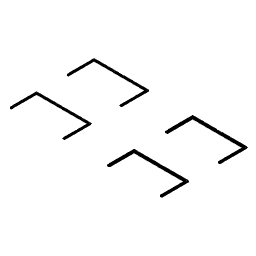
V1_V2_Panels (Autodesk Fusion 360 design; units mm, degrees)
Autodesk Fusion 360 part; units mm, degrees
note: some values were not read from the file. Chosen so that the rebuilt part matches the saved one: which bodies a step acts on; which face or edge a step refers to. Set by a fixed rule: which sketch regions a step uses.
(part 1 of 2)
sketch "Master Sketch" plane through (0, 0, 0) normal (0, 0, 1) x (1, 0, 0)
  line L0 (-121.0378, 68.2273) -> (387.1017, 68.2273)
  line L1 (389.1017, 66.2273) -> (389.1017, -187.8424)
  line L2 (-123.0378, -187.8424) -> (-123.0378, 66.2273)
  line L3 (-110.0378, -187.8424) -> (376.1017, -187.8424)
  line L4 (376.1017, -187.8424) -> (376.1017, 55.2273)
  line L5 (376.1017, 55.2273) -> (-110.0378, 55.2273)
  line L6 (-110.0378, 55.2273) -> (-110.0378, -187.8424)
  line L7 (133.0319, 68.2273) -> (133.0319, -187.8424)
  circle A0 centre (-98.0378, 64.1773) radius 3.05
  circle A1 centre (-73.0378, 58.2273) radius 1.7
  circle A2 centre (-73.0378, 58.2273) radius 2.95
  circle A3 centre (4.997, 58.2273) radius 2.95
  circle A4 centre (4.997, 58.2273) radius 1.7
  circle A5 centre (83.0319, 58.2273) radius 2.95
  circle A6 centre (83.0319, 58.2273) radius 1.7
  line L8 (153.0319, 68.2273) -> (113.0319, 68.2273) construction
  arc A7 (111.0319, 68.2273) -> (113.0319, 66.2273) centre (113.0319, 68.2273) ccw
  line L9 (113.0319, 66.2273) -> (133.0319, 66.2273)
  line L10 (153.0319, 68.2273) -> (113.0319, 68.2273) construction
  arc A8 (-121.0378, 68.2273) -> (-123.0378, 66.2273) centre (-121.0378, 66.2273) ccw
  arc A9 (389.1017, 66.2273) -> (387.1017, 68.2273) centre (387.1017, 66.2273) ccw
  line L11 (83.0319, 58.2273) -> (-73.0378, 58.2273) construction
  circle A10 centre (-143, 12) radius 3.05
  circle A11 centre (-143, -4) radius 1.7
  circle A12 centre (-143, -4) radius 2.95
  circle A13 centre (-118.9878, 43.2273) radius 3.05
  circle A14 centre (-113.0378, 18.2273) radius 1.7
  circle A15 centre (-113.0378, 18.2273) radius 2.95
  circle A16 centre (-113.0378, -59.8075) radius 1.7
  circle A17 centre (-113.0378, -59.8075) radius 2.95
  circle A18 centre (-113.0378, -137.8424) radius 1.7
  circle A19 centre (-113.0378, -137.8424) radius 2.95
  line L12 (-113.0378, 18.2273) -> (-113.0378, -137.8424) construction
  line L13 (-121.0378, -187.8424) -> (-121.0378, -167.8424)
  arc A20 (-121.0378, -167.8424) -> (-123.0378, -165.8424) centre (-123.0378, -167.8424) ccw
  line L14 (-123.0378, -187.8424) -> (-123.0378, -167.8424) construction
  line L15 (387.1017, -187.8424) -> (387.1017, -167.8424)
  line L16 (389.1017, -187.8424) -> (389.1017, -167.8424) construction
  arc A21 (389.1017, -165.8424) -> (387.1017, -167.8424) centre (389.1017, -167.8424) ccw
  circle A22 centre (379.1017, -59.8075) radius 2.95
  circle A23 centre (379.1017, -59.8075) radius 1.7
  circle A24 centre (379.1017, -137.8424) radius 1.7
  circle A25 centre (379.1017, -137.8424) radius 2.95
  circle A26 centre (379.1017, 18.2273) radius 1.7
  circle A27 centre (379.1017, 18.2273) radius 2.95
  circle A28 centre (339.1017, 58.2273) radius 1.7
  circle A29 centre (261.0668, 58.2273) radius 2.95
  arc A30 (153.0319, 66.2273) -> (155.0319, 68.2273) centre (153.0319, 68.2273) ccw
  line L17 (183.0319, 58.2273) -> (339.1017, 58.2273) construction
  circle A31 centre (183.0319, 58.2273) radius 2.95
  circle A32 centre (183.0319, 58.2273) radius 1.7
  circle A33 centre (339.1017, 58.2273) radius 2.95
  circle A34 centre (261.0668, 58.2273) radius 1.7
  line L18 (153.0319, 66.2273) -> (133.0319, 66.2273)
  line L19 (389.1017, -187.8424) -> (133.0319, -187.8424)
  line L20 (-110.0378, -187.8424) -> (-123.0378, -187.8424)
  circle A35 centre (-29.3479, 64.1773) radius 3.05
  circle A36 centre (39.342, 64.1773) radius 3.05
  circle A37 centre (-143, 12) radius 3.05
  circle A38 centre (108.0319, 64.1773) radius 3.05
  circle A39 centre (-118.9878, -25.4626) radius 3.05
  circle A40 centre (-118.9878, -94.1525) radius 3.05
  circle A41 centre (-118.9878, -162.8424) radius 3.05
  circle A42 centre (385.0517, -162.8424) radius 3.05
  circle A43 centre (385.0517, -94.1525) radius 3.05
  circle A44 centre (385.0517, -25.4626) radius 3.05
  circle A45 centre (364.1017, 64.1773) radius 3.05
  circle A46 centre (385.0517, 43.2273) radius 3.05
  circle A47 centre (226.7218, 64.1773) radius 3.05
  circle A48 centre (295.4117, 64.1773) radius 3.05
  circle A49 centre (158.0319, 64.1773) radius 3.05
  line L21 (813.9622, -187.8424) -> (1302.1017, -187.8424)
  line L22 (803.9622, 68.2273) -> (1312.1017, 68.2273)
  circle A50 centre (1310.0517, 43.2273) radius 3.05
  circle A51 centre (1083.0319, 64.1773) radius 3.05
  line L23 (1078.0319, 66.2273) -> (1058.0319, 66.2273)
  arc A52 (1078.0319, 66.2273) -> (1080.0319, 68.2273) centre (1078.0319, 68.2273) ccw
  arc A53 (803.9622, -167.8424) -> (801.9622, -165.8424) centre (801.9622, -167.8424) ccw
  circle A54 centre (1151.7218, 64.1773) radius 3.05
  circle A55 centre (806.0122, 43.2273) radius 3.05
  circle A56 centre (1220.4117, 64.1773) radius 3.05
  circle A57 centre (826.9622, 64.1773) radius 3.05
  circle A58 centre (1289.1017, 64.1773) radius 3.05
  line L24 (1301.1017, 56.2273) -> (814.9622, 56.2273)
  line L25 (1314.1017, -187.8424) -> (1058.0319, -187.8424)
  line L26 (1314.1017, 66.2273) -> (1314.1017, -187.8424)
  line L27 (813.9622, 55.2273) -> (813.9622, -187.8424)
  line L28 (1058.0319, 68.2273) -> (1058.0319, -187.8424)
  line L29 (801.9622, -187.8424) -> (801.9622, 66.2273)
  line L30 (1302.1017, -187.8424) -> (1302.1017, 55.2273)
  line L31 (1078.0319, 68.2273) -> (1038.0319, 68.2273) construction
  circle A59 centre (964.342, 64.1773) radius 3.05
  line L32 (803.9622, -187.8424) -> (803.9622, -167.8424)
  line L33 (1078.0319, 68.2273) -> (1038.0319, 68.2273) construction
  circle A60 centre (895.6521, 64.1773) radius 3.05
  circle A61 centre (1033.0319, 64.1773) radius 3.05
  line L34 (801.9622, -187.8424) -> (801.9622, -167.8424) construction
  arc A62 (1036.0319, 68.2273) -> (1038.0319, 66.2273) centre (1038.0319, 68.2273) ccw
  arc A63 (803.9622, 68.2273) -> (801.9622, 66.2273) centre (803.9622, 66.2273) ccw
  circle A64 centre (806.0122, -162.8424) radius 3.05
  circle A65 centre (806.0122, -94.1525) radius 3.05
  line L35 (813.9622, -187.8424) -> (801.9622, -187.8424)
  circle A66 centre (806.0122, -25.4626) radius 3.05
  arc A67 (1314.1017, -165.8424) -> (1312.1017, -167.8424) centre (1314.1017, -167.8424) ccw
  line L36 (1038.0319, 66.2273) -> (1058.0319, 66.2273)
  arc A68 (1314.1017, 66.2273) -> (1312.1017, 68.2273) centre (1312.1017, 66.2273) ccw
  circle A69 centre (1310.0517, -94.1525) radius 3.05
  circle A70 centre (1310.0517, -162.8424) radius 3.05
  line L37 (1312.1017, -187.8424) -> (1312.1017, -167.8424)
  circle A71 centre (1310.0517, -25.4626) radius 3.05
  line L38 (1314.1017, -187.8424) -> (1314.1017, -167.8424) construction
  arc A72 (814.9622, 56.2273) -> (813.9622, 55.2273) centre (814.9622, 55.2273) ccw
  arc A73 (1302.1017, 55.2273) -> (1301.1017, 56.2273) centre (1301.1017, 55.2273) ccw
  line L39 (821.9622, -187.8424) -> (1294.1017, -187.8424)
  line L40 (1294.1017, -187.8424) -> (1294.1017, 48.2273)
  line L41 (1294.1017, 48.2273) -> (821.9622, 48.2273)
  line L42 (821.9622, 48.2273) -> (821.9622, -187.8424)
  line L43 (376.1017, -484.7727) -> (-110.0378, -484.7727)
  circle A74 centre (385.0517, -563.7851) radius 3.05
  circle A75 centre (379.1017, -597.2913) radius 1.7
  circle A76 centre (379.1017, -672.8099) radius 2.95
  line L44 (387.1017, -722.8099) -> (387.1017, -702.8099)
  line L45 (183.0319, -481.7727) -> (339.1017, -481.7727) construction
  circle A77 centre (385.0517, -697.8099) radius 3.05
  circle A78 centre (-113.0378, -597.2913) radius 1.7
  circle A79 centre (-113.0378, -597.2913) radius 2.95
  circle A80 centre (-113.0378, -521.7727) radius 1.7
  arc A81 (-121.0378, -702.8099) -> (-123.0378, -700.8099) centre (-123.0378, -702.8099) ccw
  line L46 (-110.0378, -484.7727) -> (-110.0378, -722.8099)
  circle A82 centre (-113.0378, -521.7727) radius 2.95
  line L47 (153.0319, -471.7727) -> (113.0319, -471.7727) construction
  circle A83 centre (-118.9878, -630.7975) radius 3.05
  circle A84 centre (108.0319, -475.8227) radius 3.05
  circle A85 centre (-143, -528) radius 3.05
  circle A86 centre (-143, -544) radius 2.95
  circle A87 centre (183.0319, -481.7727) radius 1.7
  circle A88 centre (39.342, -475.8227) radius 3.05
  line L48 (-123.0378, -722.8099) -> (-123.0378, -473.7727)
  circle A89 centre (-73.0378, -481.7727) radius 2.95
  circle A90 centre (226.7218, -475.8227) radius 3.05
  circle A91 centre (158.0319, -475.8227) radius 3.05
  line L49 (-110.0378, -722.8099) -> (-123.0378, -722.8099)
  circle A92 centre (379.1017, -521.7727) radius 1.7
  circle A93 centre (-113.0378, -672.8099) radius 1.7
  circle A94 centre (379.1017, -672.8099) radius 1.7
  line L50 (389.1017, -722.8099) -> (389.1017, -702.8099) construction
  circle A95 centre (385.0517, -630.7975) radius 3.05
  line L51 (-110.0378, -722.8099) -> (376.1017, -722.8099)
  line L52 (-121.0378, -471.7727) -> (387.1017, -471.7727)
  circle A96 centre (385.0517, -496.7727) radius 3.05
  circle A97 centre (295.4117, -475.8227) radius 3.05
  circle A98 centre (261.0668, -481.7727) radius 2.95
  arc A99 (389.1017, -700.8099) -> (387.1017, -702.8099) centre (389.1017, -702.8099) ccw
  circle A100 centre (379.1017, -597.2913) radius 2.95
  circle A101 centre (364.1017, -475.8227) radius 3.05
  circle A102 centre (379.1017, -521.7727) radius 2.95
  line L53 (376.1017, -722.8099) -> (376.1017, -484.7727)
  line L54 (389.1017, -473.7727) -> (389.1017, -722.8099)
  line L55 (83.0319, -481.7727) -> (-73.0378, -481.7727) construction
  circle A103 centre (339.1017, -481.7727) radius 1.7
  line L56 (-113.0378, -521.7727) -> (-113.0378, -672.8099) construction
  circle A104 centre (339.1017, -481.7727) radius 2.95
  line L57 (389.1017, -722.8099) -> (133.0319, -722.8099)
  circle A105 centre (261.0668, -481.7727) radius 1.7
  arc A106 (389.1017, -473.7727) -> (387.1017, -471.7727) centre (387.1017, -473.7727) ccw
  line L58 (133.0319, -471.7727) -> (133.0319, -722.8099)
  arc A107 (-121.0378, -471.7727) -> (-123.0378, -473.7727) centre (-121.0378, -473.7727) ccw
  circle A108 centre (-73.0378, -481.7727) radius 1.7
  circle A109 centre (-113.0378, -672.8099) radius 2.95
  circle A110 centre (83.0319, -481.7727) radius 1.7
  circle A111 centre (-118.9878, -496.7727) radius 3.05
  circle A112 centre (83.0319, -481.7727) radius 2.95
  circle A113 centre (-118.9878, -697.8099) radius 3.05
  line L59 (113.0319, -473.7727) -> (133.0319, -473.7727)
  circle A114 centre (-143, -528) radius 3.05
  circle A115 centre (4.997, -481.7727) radius 1.7
  circle A116 centre (-143, -544) radius 1.7
  line L60 (153.0319, -471.7727) -> (113.0319, -471.7727) construction
  circle A117 centre (-118.9878, -563.7851) radius 3.05
  line L61 (-121.0378, -722.8099) -> (-121.0378, -702.8099)
  line L62 (153.0319, -473.7727) -> (133.0319, -473.7727)
  arc A118 (153.0319, -473.7727) -> (155.0319, -471.7727) centre (153.0319, -471.7727) ccw
  circle A119 centre (-98.0378, -475.8227) radius 3.05
  arc A120 (111.0319, -471.7727) -> (113.0319, -473.7727) centre (113.0319, -471.7727) ccw
  circle A121 centre (183.0319, -481.7727) radius 2.95
  circle A122 centre (4.997, -481.7727) radius 2.95
  circle A123 centre (-29.3479, -475.8227) radius 3.05
  line L63 (-123.0378, -722.8099) -> (-123.0378, -702.8099) construction
  line L64 (-118.9878, -563.7851) -> (-123.0378, -563.7851) construction
  line L65 (-123.0378, -543.7851) -> (-111.0378, -543.7851)
  line L66 (-111.0378, -543.7851) -> (-111.0378, -583.7851)
  line L67 (-111.0378, -583.7851) -> (-123.0378, -583.7851)
  line L68 (-123.0378, -583.7851) -> (-123.0378, -543.7851)
  line L69 (377.1017, -583.7851) -> (389.1017, -583.7851)
  line L70 (377.1017, -543.7851) -> (377.1017, -583.7851)
  line L71 (389.1017, -543.7851) -> (377.1017, -543.7851)
  line L72 (1302.1017, -732.8099) -> (1302.1017, -494.7727)
  line L73 (801.9622, -732.8099) -> (801.9622, -483.7727)
  line L74 (821.9622, -732.8099) -> (1294.1017, -732.8099)
  arc A124 (1302.1017, -494.7727) -> (1301.1017, -493.7727) centre (1301.1017, -494.7727) ccw
  line L75 (813.9622, -732.8099) -> (1302.1017, -732.8099)
  arc A125 (1314.1017, -483.7727) -> (1312.1017, -481.7727) centre (1312.1017, -483.7727) ccw
  line L76 (1314.1017, -732.8099) -> (1058.0319, -732.8099)
  circle A126 centre (806.0122, -506.7727) radius 3.05
  line L77 (803.9622, -481.7727) -> (1312.1017, -481.7727)
  line L78 (1301.1017, -493.7727) -> (814.9622, -493.7727)
  circle A127 centre (1083.0319, -485.8227) radius 3.05
  line L79 (1312.1017, -732.8099) -> (1312.1017, -712.8099)
  arc A128 (1036.0319, -481.7727) -> (1038.0319, -483.7727) centre (1038.0319, -481.7727) ccw
  circle A129 centre (1310.0517, -573.7851) radius 3.05
  circle A130 centre (964.342, -485.8227) radius 3.05
  circle A131 centre (1151.7218, -485.8227) radius 3.05
  circle A132 centre (1310.0517, -506.7727) radius 3.05
  circle A133 centre (1310.0517, -640.7975) radius 3.05
  line L80 (1314.1017, -732.8099) -> (1314.1017, -712.8099) construction
  line L81 (813.9622, -732.8099) -> (801.9622, -732.8099)
  circle A134 centre (806.0122, -707.8099) radius 3.05
  line L82 (813.9622, -494.7727) -> (813.9622, -732.8099)
  line L83 (801.9622, -732.8099) -> (801.9622, -712.8099) construction
  arc A135 (803.9622, -712.8099) -> (801.9622, -710.8099) centre (801.9622, -712.8099) ccw
  line L84 (1294.1017, -732.8099) -> (1294.1017, -501.7727)
  line L85 (1058.0319, -481.7727) -> (1058.0319, -732.8099)
  line L86 (1314.1017, -483.7727) -> (1314.1017, -732.8099)
  circle A136 centre (806.0122, -640.7975) radius 3.05
  circle A137 centre (806.0122, -573.7851) radius 3.05
  line L87 (1294.1017, -501.7727) -> (821.9622, -501.7727)
  line L88 (821.9622, -501.7727) -> (821.9622, -732.8099)
  line L89 (803.9622, -732.8099) -> (803.9622, -712.8099)
  circle A138 centre (826.9622, -485.8227) radius 3.05
  circle A139 centre (895.6521, -485.8227) radius 3.05
  circle A140 centre (1033.0319, -485.8227) radius 3.05
  arc A141 (1314.1017, -710.8099) -> (1312.1017, -712.8099) centre (1314.1017, -712.8099) ccw
  arc A142 (1078.0319, -483.7727) -> (1080.0319, -481.7727) centre (1078.0319, -481.7727) ccw
  line L90 (1078.0319, -481.7727) -> (1038.0319, -481.7727) construction
  arc A143 (803.9622, -481.7727) -> (801.9622, -483.7727) centre (803.9622, -483.7727) ccw
  line L91 (1078.0319, -481.7727) -> (1038.0319, -481.7727) construction
  line L92 (1038.0319, -483.7727) -> (1058.0319, -483.7727)
  circle A144 centre (1310.0517, -707.8099) radius 3.05
  circle A145 centre (1289.1017, -485.8227) radius 3.05
  line L93 (1078.0319, -483.7727) -> (1058.0319, -483.7727)
  arc A146 (814.9622, -493.7727) -> (813.9622, -494.7727) centre (814.9622, -494.7727) ccw
  circle A147 centre (1220.4117, -485.8227) radius 3.05
  line L94 (806.0122, -573.7851) -> (801.9622, -573.7851) construction
  line L95 (801.9622, -553.7851) -> (813.9622, -553.7851)
  line L96 (813.9622, -553.7851) -> (813.9622, -593.7851)
  line L97 (813.9622, -593.7851) -> (801.9622, -593.7851)
  line L98 (801.9622, -593.7851) -> (801.9622, -553.7851)
  line L99 (1314.1017, -553.7851) -> (1302.1017, -553.7851)
  line L100 (1302.1017, -553.7851) -> (1302.1017, -593.7851)
  line L101 (1302.1017, -593.7851) -> (1314.1017, -593.7851)
  circle A148 centre (-113.0378, -102.8424) radius 2.7
  circle A149 centre (379.1017, -102.8424) radius 2.7
  circle A150 centre (811.9622, -102.8424) radius 2.7
  circle A151 centre (1304.1017, -102.8424) radius 2.7
  point P0 (389.1017, 68.2273)
  point P1 (133.0319, 68.2273)
  point P2 (133.0319, 68.2273)
  point P3 (376.1017, 55.2273)
  point P4 (-123.0378, -187.8424)
  point P5 (376.1017, -187.8424)
  point P6 (389.1017, -187.8424)
  point P7 (379.1017, -137.8424)
  point P8 (379.1017, 18.2273)
  point P9 (153.0319, 68.2273)
  point P10 (1314.1017, 68.2273)
  point P11 (801.9622, -187.8424)
  point P12 (1302.1017, -187.8424)
  point P13 (1314.1017, -187.8424)
  point P14 (1058.0319, 68.2273)
  point P15 (1058.0319, 68.2273)
  point P16 (1078.0319, 68.2273)
  point P17 (389.1017, -471.7727)
  point P18 (-123.0378, -722.8099)
  point P19 (376.1017, -484.7727)
  point P20 (379.1017, -672.8099)
  point P21 (0, -540)
  point P22 (379.1017, -521.7727)
  point P23 (376.1017, -722.8099)
  point P24 (389.1017, -722.8099)
  point P25 (133.0319, -471.7727)
  point P26 (133.0319, -471.7727)
  point P27 (153.0319, -471.7727)
  point P28 (-123.0378, -563.7851)
  point P29 (801.9622, -732.8099)
  point P30 (1302.1017, -732.8099)
  point P31 (1058.0319, -481.7727)
  point P32 (1058.0319, -481.7727)
  point P33 (1078.0319, -481.7727)
  point P34 (1314.1017, -481.7727)
  point P35 (1314.1017, -732.8099)
  point P36 (801.9622, -573.7851)
  dimension "d7" = 13
  dimension "d8" = 13
  dimension "d9" = 13
  dimension "d15" = 6.1
  dimension "d19" = 4.05
  dimension "d21" = 25
  dimension "d25" = 3.4
  dimension "d26" = 5.9
  dimension "d27" = 3.4
  dimension "d28" = 5.9
  dimension "d31" = 3.4
  dimension "d32" = 5.9
  dimension "d33" = 10
  dimension "d34" = 50
  dimension "d35" = 50
  dimension "d40" = 20
  dimension "d42" = 4
  dimension "d43" = 2
  dimension "d44" = 2
  dimension "d46" = 6.1
  dimension "d47" = 3.4
  dimension "d48" = 5.9
  dimension "d49" = 6.1
  dimension "d53" = 4.05
  dimension "d57" = 25
  dimension "d58" = 3.4
  dimension "d59" = 5.9
  dimension "d60" = 3.4
  dimension "d61" = 5.9
  dimension "d62" = 3.4
  dimension "d63" = 5.9
  dimension "d64" = 50
  dimension "d65" = 10
  dimension "d66" = 50
  dimension "d67" = 256.0698
  dimension "d68" = 512.1395
  dimension "d69" = 4
  dimension "d70" = 20
  dimension "d337" = 6.1
  dimension "d338" = 93.6899
  dimension "d339" = 6.1
  dimension "d340" = 93.6899
  dimension "d341" = 6.1
  dimension "d342" = 6.1
  dimension "d343" = 25
  dimension "d344" = 6.1
  dimension "d346" = 6.1
  dimension "d348" = 6.1
  dimension "d350" = 93.6899
  dimension "d351" = 93.6899
  dimension "d352" = 25
  dimension "d353" = 2
  dimension "d354" = 2
  dimension "d355" = 12
  dimension "d356" = 12
  dimension "d357" = 12
  dimension "d358" = 6.1
  dimension "d359" = 4.05
  dimension "d360" = 25
  dimension "d370" = 20
  dimension "d371" = 4
  dimension "d372" = 2
  dimension "d373" = 2
  dimension "d377" = 6.1
  dimension "d378" = 4.05
  dimension "d379" = 25
  dimension "d389" = 256.0698
  dimension "d390" = 512.1395
  dimension "d391" = 4
  dimension "d392" = 20
  dimension "d393" = 6.1
  dimension "d394" = 93.6899
  dimension "d395" = 6.1
  dimension "d396" = 93.6899
  dimension "d398" = 6.1
  dimension "d399" = 25
  dimension "d400" = 6.1
  dimension "d401" = 6.1
  dimension "d402" = 6.1
  dimension "d403" = 93.6899
  dimension "d404" = 93.6899
  dimension "d405" = 25
  dimension "d406" = 2
  dimension "d407" = 2
  dimension "d408" = 2
  dimension "d409" = 13
  dimension "d410" = 13
  dimension "d411" = 20
  dimension "d412" = 20
  dimension "d413" = 20
  dimension "d414" = 13
  dimension "d415" = 13
  dimension "d416" = 13
  dimension "d417" = 6.1
  dimension "d418" = 4.05
  dimension "d419" = 25
  dimension "d420" = 3.4
  dimension "d421" = 5.9
  dimension "d422" = 3.4
  dimension "d423" = 5.9
  dimension "d424" = 3.4
  dimension "d425" = 5.9
  dimension "d426" = 10
  dimension "d427" = 50
  dimension "d428" = 50
  dimension "d429" = 20
  dimension "d430" = 4
  dimension "d431" = 2
  dimension "d432" = 2
  dimension "d433" = 6.1
  dimension "d434" = 3.4
  dimension "d435" = 5.9
  dimension "d436" = 6.1
  dimension "d437" = 4.05
  dimension "d438" = 25
  dimension "d439" = 3.4
  dimension "d440" = 5.9
  dimension "d441" = 3.4
  dimension "d442" = 5.9
  dimension "d443" = 3.4
  dimension "d444" = 5.9
  dimension "d445" = 50
  dimension "d446" = 10
  dimension "d447" = 50
  dimension "d448" = 251.0373
  dimension "d449" = 512.1395
  dimension "d450" = 4
  dimension "d451" = 20
  dimension "d452" = 6.1
  dimension "d453" = 93.6899
  dimension "d454" = 6.1
  dimension "d455" = 93.6899
  dimension "d456" = 6.1
  dimension "d457" = 6.1
  dimension "d458" = 25
  dimension "d459" = 6.1
  dimension "d460" = 6.1
  dimension "d461" = 6.1
  dimension "d462" = 92.0124
  dimension "d463" = 92.0124
  dimension "d464" = 25
  dimension "d465" = 2
  dimension "d466" = 2
  dimension "d467" = 12
  dimension "d468" = 40
  dimension "d469" = 12
  dimension "d470" = 12
  dimension "d471" = 12
  dimension "d472" = 6.1
  dimension "d473" = 4.05
  dimension "d474" = 25
  dimension "d484" = 20
  dimension "d485" = 4
  dimension "d486" = 2
  dimension "d487" = 2
  dimension "d488" = 6.1
  dimension "d489" = 4.05
  dimension "d490" = 25
  dimension "d500" = 251.0373
  dimension "d501" = 512.1395
  dimension "d502" = 4
  dimension "d503" = 20
  dimension "d504" = 6.1
  dimension "d505" = 93.6899
  dimension "d506" = 6.1
  dimension "d507" = 93.6899
  dimension "d508" = 6.1
  dimension "d509" = 25
  dimension "d510" = 6.1
  dimension "d511" = 6.1
  dimension "d512" = 6.1
  dimension "d513" = 92.0124
  dimension "d514" = 92.0124
  dimension "d515" = 25
  dimension "d516" = 2
  dimension "d517" = 2
  dimension "d518" = 2
  dimension "d519" = 13
  dimension "d520" = 13
  dimension "d521" = 20
  dimension "d522" = 20
  dimension "d523" = 20
  dimension "d524" = 12
  dimension "d525" = 40
  dimension "d540" = 5.4
  dimension "d541" = 85
  dimension "d542" = 5.4
  dimension "d543" = 85
  dimension "d574" = 10
  constraint horizontal L0
  constraint horizontal L19
  constraint vertical L2
  constraint horizontal L3
  constraint vertical L4
  constraint horizontal L5
  constraint coincident L3.start L19
  constraint midpoint L3 L7.end
  constraint concentric A1 A2
  constraint concentric A3 A4
  constraint concentric A5 A6
  constraint horizontal A1.centre A3.centre
  constraint horizontal A1.centre A5.centre
  constraint perpendicular L7 L8
  constraint coincident P2 P1
  constraint midpoint L8 P2
  constraint tangent A7 L9
  constraint coincident L8.end A7.centre
  constraint perpendicular L7 L10
  constraint midpoint L10 P2
  constraint coincident L0 A7.start
  constraint coincident L7 L9.end
  constraint symmetric L5.end L7 P3
  constraint coincident L0 P2
  constraint tangent L2 A8
  constraint tangent L0 A8
  constraint coincident P0 L1
  constraint coincident P0 L0
  constraint tangent L1 A9
  constraint tangent L0 A9
  constraint coincident A5.centre A6.centre
  constraint coincident A1.centre A2.centre
  constraint midpoint A3.centre L11
  constraint concentric A11 A12
  constraint concentric A14 A15
  constraint concentric A16 A17
  constraint concentric A18 A19
  constraint vertical A14.centre A16.centre
  constraint vertical A14.centre A18.centre
  constraint coincident A14.centre A15.centre
  constraint coincident A18.centre A19.centre
  constraint midpoint A16.centre L12
  constraint tangent L13 A20
  constraint perpendicular L14 L19
  constraint coincident P4 L2.start
  constraint coincident L14 P4
  constraint coincident L13.start L19
  constraint coincident L2 A20.end
  constraint symmetric P4 L7 P6
  constraint symmetric L3.start L7 P5
  constraint symmetric L7 A1 A28
  constraint symmetric L7 A2 A33
  constraint symmetric L7 A3 A29
  constraint symmetric L7 A4 A34
  constraint symmetric L7 A5 A31
  constraint symmetric L7 A6 A32
  constraint symmetric L7 L8.end P9
  constraint symmetric L7 A7.end A30.start
  constraint symmetric L7 A7 A30
  constraint symmetric L7 A7.start A30.end
  constraint symmetric L7 L9.end L18.end
  constraint symmetric L7 A5.centre L17.start
  constraint symmetric L7 A1.centre A28.centre
  constraint symmetric L7 A14 A26
  constraint symmetric L7 A15 A27
  constraint symmetric L7 A16 A23
  constraint symmetric L7 A17 A22
  constraint symmetric L7 A18 A24
  constraint symmetric L7 A19 A25
  constraint symmetric L7 A14.centre P8
  constraint symmetric L7 A18.centre P7
  constraint symmetric L7 L13.end L15.end
  constraint symmetric L7 A20 A21
  constraint symmetric L7 P4 P6
  constraint symmetric L7 L13.start L15.start
  constraint symmetric L7 A20.end A21.start
  constraint collinear L19 L20
  constraint horizontal A0.centre A35.centre
  constraint horizontal A0.centre A36.centre
  constraint horizontal A0.centre A38.centre
  constraint vertical A13.centre A39.centre
  constraint vertical A13.centre A40.centre
  constraint vertical A13.centre A41.centre
  constraint symmetric L7 A0 A45
  constraint symmetric L7 A13 A46
  constraint symmetric L7 A35 A48
  constraint symmetric L7 A36 A47
  constraint symmetric L7 A38 A49
  constraint symmetric L7 A39 A44
  constraint symmetric L7 A40 A43
  constraint symmetric L7 A41 A42
  constraint horizontal L22
  constraint horizontal L25
  constraint vertical L29
  constraint horizontal L21
  constraint vertical L30
  constraint horizontal L24
  constraint coincident L21.start L25
  constraint midpoint L25.end L21
  constraint perpendicular L28 L33
  constraint coincident P15 P14
  constraint midpoint P15 L33
  constraint tangent A62 L36
  constraint coincident L31.end L33.end
  constraint perpendicular L28 L31
  constraint midpoint P15 L31
  constraint coincident A62.start L22
  constraint coincident L23.end L28
  constraint coincident P15 L22
  constraint tangent L29 A63
  constraint tangent L22 A63
  constraint coincident P10 L26
  constraint coincident P10 L22
  constraint tangent L26 A68
  constraint tangent L22 A68
  constraint tangent A53 L32
  constraint perpendicular L25 L34
  constraint coincident P11 L29.start
  constraint coincident P11 L34
  constraint coincident L32.start L25
  constraint coincident A53.end L29
  constraint symmetric P11 P13 L28
  constraint symmetric L21.start P12 L28
  constraint symmetric L31.end P16 L28
  constraint symmetric A62.end L23.start L28
  constraint symmetric A52 L28 A62
  constraint symmetric A52.end A62.start L28
  constraint symmetric L23.end L36.end L28
  constraint symmetric A53.start A67.end L28
  constraint symmetric A53 L28 A67
  constraint symmetric L37.start L32.start L28
  constraint symmetric A67.start A53.end L28
  constraint collinear L25 L35
  constraint horizontal A60.centre A57.centre
  constraint horizontal A59.centre A57.centre
  constraint horizontal A61.centre A57.centre
  constraint vertical A66.centre A55.centre
  constraint vertical A55.centre A65.centre
  constraint vertical A55.centre A64.centre
  constraint symmetric A57 A58 L28
  constraint symmetric A50 A55 L28
  constraint symmetric A56 L28 A60
  constraint symmetric A54 L28 A59
  constraint symmetric A51 L28 A61
  constraint symmetric L28 A66 A71
  constraint symmetric L28 A65 A69
  constraint symmetric L28 A64 A70
  constraint symmetric L28 L27.start L30.end
  constraint symmetric L28 L24.end L24.start
  constraint symmetric L28 A72 A73
  constraint horizontal L39
  constraint vertical L40
  constraint horizontal L41
  constraint vertical L42
  constraint coincident L21 L39.start
  constraint horizontal L52
  constraint horizontal L57
  constraint vertical L48
  constraint horizontal L51
  constraint vertical L53
  constraint horizontal L43
  constraint coincident L46.end L57
  constraint midpoint L57.end L51
  constraint concentric A89 A108
  constraint concentric A115 A122
  constraint concentric A110 A112
  constraint horizontal A89.centre A115.centre
  constraint horizontal A89.centre L55.start
  constraint perpendicular L58 L60
  constraint coincident P26 P25
  constraint midpoint P26 L60
  constraint tangent L59 A120
  constraint coincident L47.end L60.end
  constraint perpendicular L47 L58
  constraint midpoint P26 L47
  constraint coincident A120.start L52
  constraint coincident L59.end L58
  constraint symmetric P19 L43.end L58
  constraint coincident P26 L52
  constraint tangent L48 A107
  constraint tangent L52 A107
  constraint coincident P17 L54
  constraint coincident P17 L52
  constraint tangent L54 A106
  constraint tangent L52 A106
  constraint coincident L55.start A110.centre
  constraint coincident A89.centre L55.end
  constraint midpoint A115.centre L55
  constraint concentric A86 A116
  constraint concentric A80 A82
  constraint concentric A78 A79
  constraint concentric A93 A109
  constraint vertical A80.centre A78.centre
  constraint vertical A80.centre A93.centre
  constraint coincident A80.centre A82.centre
  constraint coincident A93.centre L56.end
  constraint midpoint A78.centre L56
  constraint tangent A81 L61
  constraint perpendicular L57 L63
  constraint coincident P18 L48.start
  constraint coincident P18 L63
  constraint coincident L61.start L57
  constraint coincident A81.end L48
  constraint symmetric P18 P24 L58
  constraint symmetric L46.end P23 L58
  constraint symmetric A103 L58 A108
  constraint symmetric A89 A104 L58
  constraint symmetric A98 L58 A122
  constraint symmetric A105 L58 A115
  constraint symmetric L58 A112 A121
  constraint symmetric A87 L58 A110
  constraint symmetric L47.end P27 L58
  constraint symmetric L59.start L62.start L58
  constraint symmetric L58 A118 A120
  constraint symmetric A118.end A120.start L58
  constraint symmetric L59.end L62.end L58
  constraint symmetric L55.start L45.start L58
  constraint symmetric A89.centre L45.end L58
  constraint symmetric A80 A92 L58
  constraint symmetric A82 A102 L58
  constraint symmetric A75 A78 L58
  constraint symmetric A79 A100 L58
  constraint symmetric A93 A94 L58
  constraint symmetric A76 L58 A109
  constraint symmetric P22 A80.centre L58
  constraint symmetric P20 A93.centre L58
  constraint symmetric A81.start L44.end L58
  constraint symmetric A81 A99 L58
  constraint symmetric L44.start L61.start L58
  constraint symmetric A99.start A81.end L58
  constraint collinear L49 L57
  constraint horizontal A123.centre A119.centre
  constraint horizontal A88.centre A119.centre
  constraint horizontal A84.centre A119.centre
  constraint vertical A117.centre A111.centre
  constraint vertical A111.centre A83.centre
  constraint vertical A111.centre A113.centre
  constraint symmetric A101 L58 A119
  constraint symmetric A96 L58 A111
  constraint symmetric A97 L58 A123
  constraint symmetric A88 A90 L58
  constraint symmetric A84 A91 L58
  constraint symmetric A74 L58 A117
  constraint symmetric A83 A95 L58
  constraint symmetric A77 L58 A113
  constraint coincident A117.centre L64.start
  constraint coincident L48 P28
  constraint perpendicular L48 L64
  constraint horizontal L65
  constraint vertical L66
  constraint horizontal L67
  constraint vertical L68
  constraint midpoint L68 P28
  constraint coincident P28 L64.end
  constraint symmetric L58 L65.start L71.start
  constraint symmetric L58 L65.end L70.start
  constraint symmetric L58 L66.end L69.start
  constraint symmetric L58 L67.end L69.end
  constraint horizontal L77
  constraint horizontal L76
  constraint vertical L73
  constraint horizontal L75
  constraint vertical L72
  constraint horizontal L78
  constraint coincident L75.start L76
  constraint midpoint L76.end L75
  constraint perpendicular L85 L91
  constraint coincident P32 P31
  constraint midpoint P32 L91
  constraint tangent A128 L92
  constraint coincident A128.centre L90.end
  constraint perpendicular L85 L90
  constraint midpoint P32 L90
  constraint coincident A128.start L77
  constraint coincident L92.end L85
  constraint coincident P32 L77
  constraint tangent L73 A143
  constraint tangent L77 A143
  constraint coincident P34 L86
  constraint coincident P34 L77
  constraint tangent A125 L86
  constraint tangent A125 L77
  constraint tangent A135 L89
  constraint perpendicular L76 L83
  constraint coincident P29 L73.start
  constraint coincident P29 L83
  constraint coincident L89.start L76
  constraint coincident A135.end L73
  constraint symmetric P29 P35 L85
  constraint symmetric L75.start P30 L85
  constraint symmetric A128.centre P33 L85
  constraint symmetric A128.end A142.start L85
  constraint symmetric A128 L85 A142
  constraint symmetric A128.start A142.end L85
  constraint symmetric L92.end L93.end L85
  constraint symmetric A135.start L79.end L85
  constraint symmetric A135 L85 A141
  constraint symmetric L79.start L89.start L85
  constraint symmetric A135.end A141.start L85
  constraint collinear L76 L81
  constraint horizontal A139.centre A138.centre
  constraint horizontal A130.centre A138.centre
  constraint horizontal A140.centre A138.centre
  constraint vertical A126.centre A137.centre
  constraint vertical A136.centre A126.centre
  constraint vertical A134.centre A126.centre
  constraint symmetric L85 A138 A145
  constraint symmetric A126 A132 L85
  constraint symmetric L85 A139 A147
  constraint symmetric A130 A131 L85
  constraint symmetric A127 L85 A140
  constraint symmetric A129 L85 A137
  constraint symmetric A133 L85 A136
  constraint symmetric A134 L85 A144
  constraint symmetric L72.end L82.start L85
  constraint symmetric A124.end L78.end L85
  constraint symmetric A124 L85 A146
  constraint horizontal L74
  constraint vertical L84
  constraint horizontal L87
  constraint vertical L88
  constraint coincident L74.start L75
  constraint coincident A137.centre L94.start
  constraint coincident L73 P36
  constraint perpendicular L73 L94
  constraint horizontal L95
  constraint vertical L96
  constraint horizontal L97
  constraint vertical L98
  constraint midpoint L98 P36
  constraint coincident P36 L94.end
  constraint symmetric L85 L95.start L99.start
  constraint symmetric L85 L95.end L99.end
  constraint symmetric L85 L96.end L100.end
  constraint symmetric L85 L97.end L101.end
  constraint coincident L12 A148.centre
  constraint symmetric L7 A148 A149
  constraint symmetric L28 A150 A151
  measures "d7" distance of L2 L6
  measures "d8" distance of L1 L4
  measures "d9" distance of L0 L5
  measures "d15" diameter of A0
  measures "d19" distance of L0 A0.centre
  measures "d21" distance of L2 A0.centre
  measures "d25" diameter of A1
  measures "d26" diameter of A2
  measures "d27" diameter of A4
  measures "d28" diameter of A3
  measures "d31" diameter of A6
  measures "d32" diameter of A5
  measures "d33" distance of L0 A1.centre
  measures "d34" distance of L2 A1.centre
  measures "d35" distance of L7 A5.centre
  measures "d40" distance of L8.end P2
  measures "d42" diameter of A7
  measures "d43" radius of A8
  measures "d44" radius of A9
  measures "d46" diameter of A10
  measures "d47" diameter of A11
  measures "d48" diameter of A12
  measures "d49" diameter of A13
  measures "d53" distance of L2 A13.centre
  measures "d57" distance of L0 A13.centre
  measures "d58" diameter of A14
  measures "d59" diameter of A15
  measures "d60" diameter of A16
  measures "d61" diameter of A17
  measures "d62" diameter of A18
  measures "d63" diameter of A19
  measures "d64" distance of L0 A14.centre
  measures "d65" distance of L2 A14.centre
  measures "d66" distance of A18.centre L19
  measures "d67" distance of L0 L19
  measures "d68" distance of L1 L2
  measures "d69" diameter of A20
  measures "d70" distance of A20.centre L19
  measures "d337" diameter of A35
  measures "d338" distance of L2 A35.centre
  measures "d339" diameter of A36
  measures "d340" distance of L7 A36.centre
  measures "d341" diameter of A37
  measures "d342" diameter of A38
  measures "d343" distance of L7 A38.centre
  measures "d344" diameter of A39
  measures "d346" diameter of A40
  measures "d348" diameter of A41
  measures "d350" distance of L0 A39.centre
  measures "d351" distance of L3 A40.centre
  measures "d352" distance of L3 A41.centre
  measures "d353" distance of P4 L13.start
  measures "d354" distance of P2 L9.end
  measures "d355" distance of L27 L29
  measures "d356" distance of L26 L30
  measures "d357" distance of L22 L24
  measures "d358" diameter of A57
  measures "d359" distance of A57.centre L22
  measures "d360" distance of A57.centre L29
  measures "d370" distance of L31.end P15
  measures "d371" diameter of A62
  measures "d372" radius of A63
  measures "d373" radius of A68
  measures "d377" diameter of A55
  measures "d378" distance of A55.centre L29
  measures "d379" distance of A55.centre L22
  measures "d389" distance of L22 L25
  measures "d390" distance of L26 L29
  measures "d391" diameter of A53
  measures "d392" distance of A53.centre L25
  measures "d393" diameter of A60
  measures "d394" distance of A60.centre L29
  measures "d395" diameter of A59
  measures "d396" distance of A59.centre L28
  measures "d398" diameter of A61
  measures "d399" distance of A61.centre L28
  measures "d400" diameter of A66
  measures "d401" diameter of A65
  measures "d402" diameter of A64
  measures "d403" distance of A66.centre L22
  measures "d404" distance of A65.centre L21
  measures "d405" distance of A64.centre L21
  measures "d406" distance of P11 L32.start
  measures "d407" distance of P15 L23.end
  measures "d408" diameter of A72
  measures "d409" distance of L29 A72.centre
  measures "d410" distance of L22 A72.centre
  measures "d411" distance of L29 L42
  measures "d412" distance of L22 L41
  measures "d413" distance of L26 L40
  measures "d414" distance of L46 L48
  measures "d415" distance of L53 L54
  measures "d416" distance of L43 L52
  measures "d417" diameter of A119
  measures "d418" distance of A119.centre L52
  measures "d419" distance of A119.centre L48
  measures "d420" diameter of A108
  measures "d421" diameter of A89
  measures "d422" diameter of A115
  measures "d423" diameter of A122
  measures "d424" diameter of A110
  measures "d425" diameter of A112
  measures "d426" distance of A89.centre L52
  measures "d427" distance of A89.centre L48
  measures "d428" distance of L55.start L58
  measures "d429" distance of L47.end P26
  measures "d430" diameter of A120
  measures "d431" radius of A107
  measures "d432" radius of A106
  measures "d433" diameter of A85
  measures "d434" diameter of A116
  measures "d435" diameter of A86
  measures "d436" diameter of A111
  measures "d437" distance of A111.centre L48
  measures "d438" distance of A111.centre L52
  measures "d439" diameter of A80
  measures "d440" diameter of A82
  measures "d441" diameter of A78
  measures "d442" diameter of A79
  measures "d443" diameter of A93
  measures "d444" diameter of A109
  measures "d445" distance of A80.centre L52
  measures "d446" distance of A80.centre L48
  measures "d447" distance of A93.centre L57
  measures "d448" distance of L52 L57
  measures "d449" distance of L48 L54
  measures "d450" diameter of A81
  measures "d451" distance of A81.centre L57
  measures "d452" diameter of A123
  measures "d453" distance of A123.centre L48
  measures "d454" diameter of A88
  measures "d455" distance of A88.centre L58
  measures "d456" diameter of A114
  measures "d457" diameter of A84
  measures "d458" distance of A84.centre L58
  measures "d459" diameter of A117
  measures "d460" diameter of A83
  measures "d461" diameter of A113
  measures "d462" distance of A117.centre L52
  measures "d463" distance of A83.centre L51
  measures "d464" distance of A113.centre L51
  measures "d465" distance of P18 L61.start
  measures "d466" distance of P26 L59.end
  measures "d467" distance of L65.start L65.end
  measures "d468" distance of L65.start L67.end
  measures "d469" distance of L73 L82
  measures "d470" distance of L72 L86
  measures "d471" distance of L77 L78
  measures "d472" diameter of A138
  measures "d473" distance of A138.centre L77
  measures "d474" distance of A138.centre L73
  measures "d484" distance of P32 A128.centre
  measures "d485" diameter of A128
  measures "d486" radius of A143
  measures "d487" radius of A125
  measures "d488" diameter of A126
  measures "d489" distance of A126.centre L73
  measures "d490" distance of A126.centre L77
  measures "d500" distance of L76 L77
  measures "d501" distance of L73 L86
  measures "d502" diameter of A135
  measures "d503" distance of L83.end L76
  measures "d504" diameter of A139
  measures "d505" distance of A139.centre L73
  measures "d506" diameter of A130
  measures "d507" distance of A130.centre L85
  measures "d508" diameter of A140
  measures "d509" distance of A140.centre L85
  measures "d510" diameter of A137
  measures "d511" diameter of A136
  measures "d512" diameter of A134
  measures "d513" distance of A137.centre L77
  measures "d514" distance of A136.centre L75
  measures "d515" distance of A134.centre L75
  measures "d516" distance of P29 L89.start
  measures "d517" distance of L92.end P32
  measures "d518" diameter of A146
  measures "d519" distance of A146.centre L73
  measures "d520" distance of A146.centre L77
  measures "d521" distance of L73 L88
  measures "d522" distance of L77 L87
  measures "d523" distance of L84 L86
  measures "d524" distance of L95.start L95.end
  measures "d525" distance of L95.start L97.end
  measures "d540" diameter of A148
  measures "d541" distance of L3 A148.centre
  measures "d542" diameter of A150
  measures "d543" distance of L39 A150.centre
  measures "d574" distance of L29 A150.centre
extrude "Extrude7" add sketch "Master Sketch" against normal blind 4 contours L0 L2 L5 L6 L7 A7 L9 A8 L13 A20 L20 | L0 L7 A7 L9 | L0 L7 A30 L18 | L2 L13 A20 L20 | L0 L1 L4 L5 L7 A9 L15 A21 A30 L18 L19 | L3 L5 L6 L7 | L3 L4 L5 L7 L19 | L1 L15 A21 L19 | A0 | A1 | A2 | A3 | A4 | A5 | A6 | A13 | A14 | A15 | A16 | A17 | A18 | A19 | A22 | A23 | A24 | A25 | A26 | A27 | A28 | A29 | A31 | A32 | A33 | A34 | A35 | A36 | A38 | A39 | A40 | A41 | A42 | A43 | A44 | A45 | A46 | A47 | A48 | A49 | A148 | A149 makes body 1 in component "Top_Panel"
extrude "Extrude8" cut sketch "Master Sketch" against normal blind 50 contours L3 L5 L6 L7 | L3 L4 L5 L7 L19 | A1 | A4 | A6 | A14 | A16 | A18 | A23 | A24 | A26 | A28 | A32 | A34 bodies 1 in component "Top_Panel"
extrude "Extrude9" cut sketch "Master Sketch" against normal blind 3.1 contours A2 | A3 | A5 | A15 | A17 | A19 | A22 | A25 | A27 | A29 | A31 | A33 bodies 1 in component "Top_Panel"
extrude "Extrude10" cut sketch "Master Sketch" against normal blind 3.1 contours A0 | A13 | A35 | A36 | A38 | A39 | A40 | A41 | A42 | A43 | A44 | A45 | A46 | A47 | A48 | A49 bodies 1 in component "Top_Panel"
revolve "Revolve4" cut sketch "Master Sketch" angle 360 about axis through (-123.0378, -187.8424, 0) along (0, 1, 0) contours L2 L13 A20 L20 bodies 1 in component "Top_Panel"
revolve "Revolve5" cut sketch "Master Sketch" angle 360 about axis through (-121.0378, 68.2273, 0) along (1, 0, 0) contours L0 L7 A7 L9 | L0 L7 A30 L18 bodies 1 in component "Top_Panel"
revolve "Revolve6" cut sketch "Master Sketch" angle 360 about axis through (389.1017, 66.2273, 0) along (0, -1, 0) contours L1 L15 A21 L19 bodies 1 in component "Top_Panel"
sketch "Sketch1" plane through (0, 0, 0) normal (0, 0, 1) x (-1, 0, 0) in component "Top_Panel"
  arc A0 (-389.1017, 165.8424) -> (-387.1017, 167.8424) centre (-389.1017, 167.8424) ccw
  line L0 (-389.1017, 165.8424) -> (-389.1017, -66.2273)
  arc A1 (-389.1017, -66.2273) -> (-387.1017, -68.2273) centre (-387.1017, -66.2273) ccw
  line L1 (-387.1017, -68.2273) -> (-155.0319, -68.2273)
  arc A2 (-153.0319, -66.2273) -> (-155.0319, -68.2273) centre (-153.0319, -68.2273) ccw
  line L2 (-153.0319, -66.2273) -> (-113.0319, -66.2273)
  arc A3 (-111.0319, -68.2273) -> (-113.0319, -66.2273) centre (-113.0319, -68.2273) ccw
  line L3 (-111.0319, -68.2273) -> (121.0378, -68.2273)
  arc A4 (121.0378, -68.2273) -> (123.0378, -66.2273) centre (121.0378, -66.2273) ccw
  line L4 (123.0378, -66.2273) -> (123.0378, 165.8424)
  arc A5 (121.0378, 167.8424) -> (123.0378, 165.8424) centre (123.0378, 167.8424) ccw
  line L5 (121.0378, 167.8424) -> (121.0378, 187.8424)
  line L6 (121.0378, 187.8424) -> (110.0378, 187.8424)
  line L7 (110.0378, 187.8424) -> (110.0378, -55.2273)
  line L8 (110.0378, -55.2273) -> (-376.1017, -55.2273)
  line L9 (-376.1017, -55.2273) -> (-376.1017, 187.8424)
  line L10 (-376.1017, 187.8424) -> (-387.1017, 187.8424)
  line L11 (-387.1017, 187.8424) -> (-387.1017, 167.8424)
  circle A6 centre (-379.1017, 137.8424) radius 2.95
  circle A7 centre (-261.0668, -58.2273) radius 2.95
  circle A8 centre (73.0378, -58.2273) radius 2.95
  circle A9 centre (113.0378, 137.8424) radius 2.95
  circle A10 centre (-4.997, -58.2273) radius 2.95
  circle A11 centre (-339.1017, -58.2273) radius 2.95
  circle A12 centre (-379.1017, 59.8075) radius 2.95
  circle A13 centre (-183.0319, -58.2273) radius 2.95
  circle A14 centre (113.0378, -18.2273) radius 2.95
  circle A15 centre (113.0378, 59.8075) radius 2.95
  circle A16 centre (-83.0319, -58.2273) radius 2.95
  circle A17 centre (-379.1017, -18.2273) radius 2.95
  circle A18 centre (118.9878, 162.8424) radius 3.05
  circle A19 centre (98.0378, -64.1773) radius 3.05
  circle A20 centre (-158.0319, -64.1773) radius 3.05
  circle A21 centre (-385.0517, -43.2273) radius 3.05
  circle A22 centre (-385.0517, 162.8424) radius 3.05
  circle A23 centre (-364.1017, -64.1773) radius 3.05
  circle A24 centre (-108.0319, -64.1773) radius 3.05
  circle A25 centre (118.9878, -43.2273) radius 3.05
  circle A26 centre (118.9878, 94.1525) radius 3.05
  circle A27 centre (29.3479, -64.1773) radius 3.05
  circle A28 centre (-226.7218, -64.1773) radius 3.05
  circle A29 centre (-385.0517, 25.4626) radius 3.05
  circle A30 centre (-385.0517, 94.1525) radius 3.05
  circle A31 centre (-295.4117, -64.1773) radius 3.05
  circle A32 centre (-39.342, -64.1773) radius 3.05
  circle A33 centre (118.9878, 25.4626) radius 3.05
  line L12 (-133.0319, -68.2136) -> (-133.0319, -55.2273)
  constraint midpoint L8 L12.end
  constraint perpendicular L8 L12
split "Split1" by curves path "Sketch1" along L12 bodies 1 makes body 2 at (-115.4304, -171.7393, -4) in component "Top_Panel"
chamfer "Chamfer2" distance 0.4 angle 45 2 edges at (143.0319, 66.2273, 0) (154.4461, 66.8131, 0) 1 faces at (-115.4304, -171.7393, -4) on bodies 1 2 in component "Top_Panel"
chamfer "Chamfer3" distance 0.4 angle 45 1 faces at (381.6101, -171.7147, -4) on bodies 1 in component "Top_Panel"
chamfer "Chamfer4" distance 0.1 angle 45 28 edges at (-121.8314, -161.7395, 0) (-115.7882, -136.7757, 0) (-121.8314, -93.0496, 0) (-115.7882, -58.7408, 0) (-121.8314, -24.3597, 0) (-115.7882, 19.2941, 0) (-121.8314, 44.3303, 0) (-100.8814, 65.2803, 0) (-75.7882, 59.2941, 0) (-32.1915, 65.2803, 0) (2.2467, 59.2941, 0) (36.4984, 65.2803, 0) (80.2815, 59.2941, 0) (105.1883, 65.2803, 0) (180.2815, 59.2941, 0) (155.1883, 65.2803, 0) (223.8782, 65.2803, 0) (292.5681, 65.2803, 0) (258.3164, 59.2941, 0) (336.3513, 59.2941, 0) (361.2581, 65.2803, 0) (382.2081, 44.3303, 0) (376.3513, 19.2941, 0) (382.2081, -24.3597, 0) (376.3513, -58.7408, 0) (382.2081, -93.0496, 0) (376.3513, -136.7757, 0) (382.2081, -161.7395, 0) on bodies 1 2 in component "Top_Panel"
extrude "Extrude1" add sketch "Master Sketch" against normal blind 4 separate body contours L43 L51 L53 L57 L58 | L43 L44 L52 A99 L53 L54 L57 A106 L58 L62 A118 L69 L70 L71 | L43 L46 L51 L58 | L43 A81 L46 L48 L49 L52 L58 A107 L59 L61 A120 L65 L66 L67 | L52 L58 L59 A120 | L52 L58 L62 A118 | L44 A99 L54 L57 | A81 L48 L49 L61 | L54 L69 L70 L71 | L48 L65 L66 L67 L68 | A74 | A75 | A76 | A77 | A78 | A79 | A80 | A82 | A83 | A84 | A87 | A88 | A89 | A90 | A91 | A92 | A93 | A94 | A95 | A96 | A97 | A98 | A100 | A101 | A102 | A103 | A104 | A105 | A108 | A109 | A110 | A111 | A112 | A113 | A115 | A117 | A119 | A121 | A122 | A123 makes body 3 in component "Side_Panel"
extrude "Extrude2" cut sketch "Master Sketch" against normal blind 21 contours L43 L51 L53 L57 L58 | L43 L46 L51 L58 | A75 | A78 | A80 | A87 | A92 | A93 | A94 | A103 | A105 | A108 | A110 | A115 bodies 3 in component "Side_Panel"
extrude "Extrude3" cut sketch "Master Sketch" against normal blind 3.1 contours A76 | A79 | A82 | A89 | A98 | A100 | A102 | A104 | A109 | A112 | A115 | A121 | A122 bodies 3 in component "Side_Panel"
extrude "Extrude4" cut sketch "Master Sketch" against normal blind 3.1 contours A74 | A77 | A83 | A84 | A88 | A90 | A91 | A95 | A96 | A97 | A101 | A111 | A113 | A117 | A119 | A123 bodies 3 in component "Side_Panel"
revolve "Revolve1" cut sketch "Master Sketch" angle 360 about axis through (-123.0378, -722.8099, 0) along (0, 1, 0) contours A81 L48 L49 L61 bodies 3 in component "Side_Panel"
revolve "Revolve2" cut sketch "Master Sketch" angle 360 about axis through (-121.0378, -471.7727, 0) along (1, 0, 0) contours L52 L58 L59 A120 | L52 L58 L62 A118 bodies 3 in component "Side_Panel"
revolve "Revolve3" cut sketch "Master Sketch" angle 360 about axis through (389.1017, -473.7727, 0) along (0, -1, 0) contours L44 A99 L54 L57 bodies 3 in component "Side_Panel"
chamfer "Chamfer1" distance 0.1 angle 45 26 edges at (-121.8314, -696.707, 0) (-115.7882, -671.7432, 0) (-121.8314, -629.6946, 0) (-115.7882, -596.2245, 0) (-121.8314, -562.6822, 0) (-115.7882, -520.7059, 0) (-121.8314, -495.6697, 0) (-100.8814, -474.7197, 0) (-32.1915, -474.7197, 0) (-75.7882, -480.7059, 0) (36.4984, -474.7197, 0) (80.2815, -480.7059, 0) (105.1883, -474.7197, 0) (155.1883, -474.7197, 0) (180.2815, -480.7059, 0) (223.8782, -474.7197, 0) (258.3164, -480.7059, 0) (292.5681, -474.7197, 0) (336.3513, -480.7059, 0) (361.2581, -474.7197, 0) (382.2081, -495.6697, 0) (376.3513, -520.7059, 0) (382.2081, -562.6822, 0) (376.3513, -596.2245, 0) (376.3513, -671.7432, 0) (382.2081, -696.707, 0) on bodies 3 in component "Side_Panel"